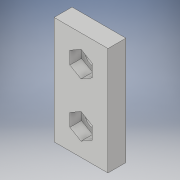
# Autodesk Inventor part: КВ33.044.002 - ограничитель перемещения по оси Z
Saved by Autodesk Inventor 2019 (Build 230136000, 136)
## iProperties
Created: 2019-11-29
Part Number: КВ33.044.002 - ограничитель перемещения по оси Z
Material: Типовые
Document SubType Name: Modeling
Designer: Петров Иван
Density: 1 g/cm^3
Appearance: По умолчанию
Author: Петров Иван
Autodesk Inventor part; units mm, degrees
(part 1 of 2)
ref_plane "YZ Plane" through (0, 0, 0) normal (1, 0, 0) x (0, 1, 0)
ref_plane "XZ Plane" through (0, 0, 0) normal (0, 1, 0) x (-1, 0, 0)
ref_plane "XY Plane" through (0, 0, 0) normal (0, 0, 1) x (1, 0, 0)
sketch "Эскиз1" plane through (0, 0, 0) normal (0, 0, 1) x (1, 0, 0)
  line L0 (-15, -30) -> (15, -30)
  line L1 (15, -30) -> (15, 30)
  line L2 (15, 30) -> (-15, 30)
  line L3 (-15, 30) -> (-15, -30)
  line L4 (-15, -30) -> (15, 30) construction
  line L5 (15, -30) -> (-15, 30) construction
  line L6 (0, 0) -> (0, 15)
  circle A0 centre (0, 15) radius 4.1
  line L7 (0, 0) -> (0, -15)
  circle A1 centre (0, -15) radius 4.1
  dimension "d0" = 30
  dimension "d1" = 60
  dimension "d2" = 15
  dimension "d3" = 8.2
  dimension "d4" = 15
  dimension "d5" = 8.2
  constraints: 16 end point, 2 centre point, 2 coincident, 2 midpoint, 2 parallel, 2 vertical, 1 horizontal, 1 perpendicular
  measures "d0" distance of L2.end L1.end
  measures "d1" distance of L1.end L0.end
  measures "d2" distance of L6.start L6.end
  measures "d3" diameter of A0
  measures "d4" distance of L6.start L7.end
  measures "d5" diameter of A1
extrude "Выдавливание1" add sketch "Эскиз1" along normal blind 10
sketch "Эскиз2" plane through (0, 0, 10) normal (0, 0, 1) x (1, 0, 0)
  circle A0 centre (0, 15) radius 4.1 projected
  line L0 (0, 22.15) -> (6.1921, 18.575)
  line L1 (6.1921, 18.575) -> (6.1921, 11.425)
  line L2 (6.1921, 11.425) -> (0, 7.85)
  line L3 (0, 7.85) -> (-6.1921, 11.425)
  line L4 (-6.1921, 11.425) -> (-6.1921, 18.575)
  line L5 (-6.1921, 18.575) -> (0, 22.15)
  point P0 (0, 0)
  dimension "d8" = 14.3
  constraints: 12 end point, 1 coincident, 13 other
  measures "d8" distance of L2.end L0.start
extrude "Выдавливание2" cut sketch "Эскиз2" against normal blind 6.5
mirror "Зеркальное отражение1" about plane through (0, 0, 0) normal (0, 1, 0) of "Выдавливание2"
sketch "Эскиз3" plane through (15, -30, 0) normal (1, 0, 0) x (0, 0, -1)
  arc A0 (-20.0782, 47.7916) -> (-19.9782, 47.8916) centre (-20.0782, 47.8916) ccw
  line L0 (-19.9782, 47.8916) -> (-19.9782, 57.5416)
  arc A1 (-19.9782, 57.5416) -> (-20.0782, 57.6416) centre (-20.0782, 57.5416) ccw
  line L1 (-19.8782, 57.6416) -> (-19.3657, 57.6416)
  line L2 (-19.3657, 57.6416) -> (-19.274, 56.2076)
  arc A2 (-19.274, 56.2076) -> (-15.0825, 56.2076) centre (-17.1782, 56.3416) ccw
  line L3 (-15.0825, 56.2076) -> (-14.9908, 57.6416)
  line L4 (-14.9908, 57.6416) -> (-10.7025, 57.6416)
  arc A3 (-10.6318, 57.6123) -> (-10.7025, 57.6416) centre (-10.7025, 57.5416) ccw
  line L5 (-10.6318, 57.6123) -> (-10.3075, 57.288)
  arc A4 (-10.3075, 57.288) -> (-9.954, 57.1416) centre (-9.954, 57.6416) ccw
  line L6 (-9.954, 57.1416) -> (-0.2782, 57.1416)
  arc A5 (-0.1782, 57.0416) -> (-0.2782, 57.1416) centre (-0.2782, 57.0416) ccw
  line L7 (-0.1782, 57.0416) -> (-0.1782, 47.8916)
  arc A6 (-0.2782, 47.7916) -> (-0.1782, 47.8916) centre (-0.2782, 47.8916) ccw
  line L8 (-0.2782, 47.7916) -> (-3.204, 47.7916)
  arc A7 (-3.204, 47.7916) -> (-3.5575, 47.6451) centre (-3.204, 47.2916) ccw
  line L9 (-3.5575, 47.6451) -> (-3.8818, 47.3209)
  arc A8 (-3.9525, 47.2916) -> (-3.8818, 47.3209) centre (-3.9525, 47.3916) ccw
  line L10 (-3.9525, 47.2916) -> (-6.704, 47.2916)
  arc A9 (-6.7747, 47.3209) -> (-6.704, 47.2916) centre (-6.704, 47.3916) ccw
  line L11 (-6.7747, 47.3209) -> (-7.099, 47.6451)
  arc A10 (-7.099, 47.6451) -> (-7.4525, 47.7916) centre (-7.4525, 47.2916) ccw
  line L12 (-7.4525, 47.7916) -> (-12.704, 47.7916)
  arc A11 (-12.704, 47.7916) -> (-13.0575, 47.6451) centre (-12.704, 47.2916) ccw
  line L13 (-13.0575, 47.6451) -> (-13.3818, 47.3209)
  arc A12 (-13.4525, 47.2916) -> (-13.3818, 47.3209) centre (-13.4525, 47.3916) ccw
  line L14 (-13.4525, 47.2916) -> (-16.204, 47.2916)
  arc A13 (-16.2747, 47.3209) -> (-16.204, 47.2916) centre (-16.204, 47.3916) ccw
  line L15 (-16.2747, 47.3209) -> (-16.599, 47.6451)
  arc A14 (-16.599, 47.6451) -> (-16.9525, 47.7916) centre (-16.9525, 47.2916) ccw
  line L16 (-16.9525, 47.7916) -> (-19.8782, 47.7916)
  arc A15 (-19.9782, 47.8916) -> (-19.8782, 47.7916) centre (-19.8782, 47.8916) ccw
  arc A16 (-19.8782, 57.6416) -> (-19.9782, 57.5416) centre (-19.8782, 57.5416) ccw
  circle A17 centre (-14.8282, 49.8416) radius 1.25
  circle A18 centre (-5.3282, 49.8416) radius 1.25
  line L17 (-4.1549, 52.0916) -> (-4.7716, 53.3916)
  line L18 (-4.7716, 53.3916) -> (-4.7882, 53.3916)
  line L19 (-4.7882, 53.3916) -> (-5.3882, 52.0916)
  line L20 (-5.3882, 52.0916) -> (-5.2614, 52.0916)
  line L21 (-5.2614, 52.0916) -> (-5.0692, 52.5083)
  line L22 (-5.0692, 52.5083) -> (-4.4799, 52.5083)
  line L23 (-4.4799, 52.5083) -> (-4.2823, 52.0916)
  line L24 (-4.2823, 52.0916) -> (-4.1549, 52.0916)
  spline S0 degree 3 poles (-6.9749, 53.028) (-6.9747, 53.0369) (-6.9742, 53.0544) (-6.9701, 53.08) (-6.9639, 53.1048) (-6.955, 53.1286) (-6.9433, 53.1515) (-6.929, 53.1732) (-6.9125, 53.1943) (-6.8934, 53.214) (-6.8725, 53.2321) (-6.8503, 53.2481) (-6.8269, 53.2615) (-6.8023, 53.2725) (-6.7766, 53.2811) (-6.7497, 53.2871) (-6.7217, 53.2908) (-6.7026, 53.2913) (-6.6929, 53.2916) knots 0 0 0 0 0.061965 0.122122 0.180988 0.239933 0.299906 0.359989 0.421776 0.486576 0.551535 0.615018 0.677259 0.73973 0.80305 0.866495 0.931973 1 1 1 1
  spline S1 degree 3 poles (-6.6929, 53.2916) (-6.6827, 53.2913) (-6.6627, 53.2908) (-6.6334, 53.2872) (-6.6055, 53.2809) (-6.5788, 53.2722) (-6.5533, 53.2613) (-6.5292, 53.2477) (-6.5066, 53.2314) (-6.4852, 53.213) (-6.4656, 53.1924) (-6.4484, 53.1696) (-6.4333, 53.1447) (-6.4201, 53.1181) (-6.4095, 53.0892) (-6.4013, 53.0584) (-6.3948, 53.0257) (-6.3927, 53.0032) (-6.3916, 52.9916) knots 0 0 0 0 0.064439 0.126547 0.186887 0.245878 0.304041 0.362191 0.420976 0.48066 0.5406 0.600689 0.661936 0.724443 0.789038 0.856314 0.926352 1 1 1 1
  line L25 (-6.3916, 52.9916) -> (-6.2749, 52.9916)
  spline S2 degree 3 poles (-6.2749, 52.9916) (-6.2757, 53.0071) (-6.2772, 53.0375) (-6.2842, 53.0818) (-6.2942, 53.1241) (-6.3083, 53.1642) (-6.3259, 53.2023) (-6.347, 53.2384) (-6.3719, 53.2722) (-6.4002, 53.3034) (-6.431, 53.3321) (-6.4641, 53.3568) (-6.499, 53.3778) (-6.5354, 53.3952) (-6.5738, 53.4084) (-6.6139, 53.4181) (-6.6558, 53.424) (-6.6843, 53.4246) (-6.6989, 53.4249) knots 0 0 0 0 0.068791 0.135103 0.198979 0.261904 0.323495 0.385195 0.446969 0.509765 0.572251 0.633405 0.693251 0.752583 0.812579 0.873275 0.93555 1 1 1 1
  spline S3 degree 3 poles (-6.6989, 53.4249) (-6.7131, 53.4246) (-6.7411, 53.4239) (-6.782, 53.4183) (-6.8209, 53.4095) (-6.8578, 53.3971) (-6.8924, 53.3805) (-6.9248, 53.3605) (-6.9556, 53.3374) (-6.9833, 53.3102) (-7.0088, 53.2811) (-7.0307, 53.2501) (-7.0495, 53.2181) (-7.0652, 53.1848) (-7.0767, 53.1499) (-7.0855, 53.114) (-7.0904, 53.0766) (-7.0912, 53.0513) (-7.0916, 53.0385) knots 0 0 0 0 0.069475 0.136517 0.200789 0.26383 0.325735 0.387291 0.449509 0.512968 0.576275 0.63758 0.697903 0.757172 0.816599 0.876653 0.93729 1 1 1 1
  spline S4 degree 3 poles (-7.0916, 53.0385) (-7.0909, 53.0204) (-7.0897, 52.9845) (-7.079, 52.9317) (-7.0624, 52.8806) (-7.0423, 52.8395) (-7.0221, 52.8063) (-7.0039, 52.779) (-6.9825, 52.7497) (-6.9577, 52.7183) (-6.9301, 52.6847) (-6.8992, 52.6488) (-6.865, 52.6111) (-6.841, 52.5854) (-6.8286, 52.5721) knots 0 0 0 0 0.098702 0.195672 0.292422 0.391343 0.444462 0.504229 0.570352 0.642546 0.722288 0.807921 0.90047 1 1 1 1
  line L26 (-6.8286, 52.5721) -> (-6.5033, 52.2249)
  line L27 (-6.5033, 52.2249) -> (-7.1082, 52.2249)
  line L28 (-7.1082, 52.2249) -> (-7.1082, 52.0916)
  line L29 (-7.1082, 52.0916) -> (-6.2249, 52.0916)
  line L30 (-6.2249, 52.0916) -> (-6.7291, 52.6296)
  spline S5 degree 3 poles (-6.7291, 52.6296) (-6.7413, 52.6424) (-6.7649, 52.667) (-6.7983, 52.703) (-6.8282, 52.7363) (-6.855, 52.767) (-6.8779, 52.7954) (-6.8983, 52.8208) (-6.9147, 52.8441) (-6.9324, 52.8711) (-6.9495, 52.9041) (-6.9643, 52.9444) (-6.9733, 52.9859) (-6.9744, 53.0139) (-6.9749, 53.028) knots 0 0 0 0 0.110803 0.212829 0.306101 0.390647 0.466924 0.534481 0.593587 0.644557 0.7362 0.825024 0.911986 1 1 1 1
  line L31 (-7.4849, 52.7416) -> (-7.6182, 53.3916)
  line L32 (-7.6182, 53.3916) -> (-8.1516, 53.3916)
  line L33 (-8.1516, 53.3916) -> (-8.1516, 53.2583)
  line L34 (-8.1516, 53.2583) -> (-7.7094, 53.2583)
  line L35 (-7.7094, 53.2583) -> (-7.6393, 52.9163)
  spline S6 degree 3 poles (-7.6393, 52.9163) (-7.6531, 52.9201) (-7.6798, 52.9275) (-7.7191, 52.9357) (-7.7565, 52.9406) (-7.7807, 52.9413) (-7.7925, 52.9416) knots 0 0 0 0 0.275068 0.532901 0.773973 1 1 1 1
  spline S7 degree 3 poles (-7.7925, 52.9416) (-7.807, 52.9413) (-7.8355, 52.9407) (-7.8773, 52.9347) (-7.9171, 52.9254) (-7.955, 52.9123) (-7.991, 52.8957) (-8.0247, 52.8748) (-8.0567, 52.8505) (-8.0864, 52.8225) (-8.1134, 52.7917) (-8.1371, 52.7586) (-8.1572, 52.7235) (-8.1734, 52.686) (-8.1863, 52.6467) (-8.1949, 52.605) (-8.2006, 52.5614) (-8.2012, 52.5315) (-8.2016, 52.5163) knots 0 0 0 0 0.065808 0.129394 0.190894 0.251281 0.310815 0.370371 0.430768 0.492881 0.555104 0.616067 0.677256 0.73826 0.800762 0.864778 0.931045 1 1 1 1
  spline S8 degree 3 poles (-8.2016, 52.5163) (-8.2013, 52.5057) (-8.2008, 52.4847) (-8.1983, 52.4534) (-8.1935, 52.4228) (-8.1871, 52.3929) (-8.1787, 52.3637) (-8.1686, 52.3351) (-8.1562, 52.3073) (-8.1426, 52.2801) (-8.1272, 52.254) (-8.1102, 52.2296) (-8.0923, 52.2066) (-8.0729, 52.1851) (-8.0521, 52.1653) (-8.0299, 52.1471) (-8.0066, 52.1302) (-7.9819, 52.1153) (-7.9562, 52.1016) (-7.9292, 52.0903) (-7.9016, 52.0802) (-7.8728, 52.0722) (-7.8431, 52.0659) (-7.8123, 52.0617) (-7.7805, 52.0585) (-7.759, 52.0584) (-7.7482, 52.0583) knots 0 0 0 0 0.044014 0.087434 0.130118 0.172554 0.214555 0.256298 0.298438 0.340849 0.382715 0.423924 0.464246 0.504074 0.543862 0.583567 0.623094 0.663229 0.703551 0.743938 0.784541 0.82575 0.867757 0.910745 0.954914 1 1 1 1
  spline S9 degree 3 poles (-7.7482, 52.0583) (-7.7352, 52.0585) (-7.7098, 52.059) (-7.6724, 52.0643) (-7.6365, 52.0719) (-7.6023, 52.0832) (-7.5694, 52.0975) (-7.5385, 52.1155) (-7.5085, 52.1359) (-7.4808, 52.16) (-7.4552, 52.1864) (-7.4322, 52.215) (-7.4117, 52.2453) (-7.3941, 52.2776) (-7.379, 52.3117) (-7.3672, 52.3478) (-7.3577, 52.3856) (-7.3536, 52.4117) (-7.3516, 52.4249) knots 0 0 0 0 0.065421 0.128708 0.190236 0.250724 0.310637 0.370766 0.431615 0.493523 0.555883 0.617342 0.678668 0.740711 0.802985 0.866803 0.932347 1 1 1 1
  line L36 (-7.3516, 52.4249) -> (-7.4682, 52.4249)
  spline S10 degree 3 poles (-7.4682, 52.4249) (-7.4711, 52.4125) (-7.4766, 52.3887) (-7.4887, 52.3552) (-7.5035, 52.3254) (-7.5212, 52.2988) (-7.5422, 52.2756) (-7.5661, 52.255) (-7.593, 52.2363) (-7.6229, 52.2208) (-7.6544, 52.2075) (-7.6873, 52.1987) (-7.7209, 52.1925) (-7.7436, 52.1919) (-7.755, 52.1916) knots 0 0 0 0 0.094687 0.181994 0.264377 0.34218 0.418618 0.496509 0.577369 0.661511 0.746733 0.831258 0.915206 1 1 1 1
  spline S11 degree 3 poles (-7.755, 52.1916) (-7.7661, 52.1919) (-7.788, 52.1925) (-7.8202, 52.1971) (-7.8514, 52.2042) (-7.8811, 52.2149) (-7.9099, 52.2278) (-7.9371, 52.2444) (-7.9634, 52.2635) (-7.9881, 52.2854) (-8.0107, 52.3096) (-8.0306, 52.3354) (-8.0473, 52.3629) (-8.0613, 52.3917) (-8.0719, 52.422) (-8.0795, 52.4538) (-8.084, 52.487) (-8.0846, 52.5097) (-8.0849, 52.5213) knots 0 0 0 0 0.064207 0.126425 0.18768 0.248216 0.308305 0.369661 0.431699 0.495947 0.559758 0.622295 0.683911 0.745092 0.80674 0.869087 0.93329 1 1 1 1
  spline S12 degree 3 poles (-8.0849, 52.5213) (-8.0847, 52.5317) (-8.0842, 52.5521) (-8.0803, 52.582) (-8.0735, 52.6102) (-8.064, 52.637) (-8.052, 52.6624) (-8.0374, 52.6863) (-8.0198, 52.7085) (-7.9997, 52.7289) (-7.9777, 52.7478) (-7.9534, 52.7639) (-7.9273, 52.7775) (-7.8997, 52.7891) (-7.87, 52.7975) (-7.8388, 52.8038) (-7.8057, 52.8075) (-7.783, 52.808) (-7.7714, 52.8083) knots 0 0 0 0 0.065351 0.127916 0.18836 0.247216 0.30563 0.36377 0.422661 0.482687 0.5433 0.604118 0.664965 0.727413 0.791468 0.858055 0.927037 1 1 1 1
  spline S13 degree 3 poles (-7.7714, 52.8083) (-7.7613, 52.808) (-7.7405, 52.8076) (-7.7086, 52.8043) (-7.675, 52.799) (-7.64, 52.7917) (-7.6034, 52.7822) (-7.5652, 52.7708) (-7.5255, 52.7572) (-7.4987, 52.7469) (-7.4849, 52.7416) knots 0 0 0 0 0.102203 0.211023 0.3251 0.446502 0.573788 0.708901 0.850358 1 1 1 1
  line L37 (-10.9316, 52.0916) -> (-11.5482, 53.3916)
  line L38 (-11.5482, 53.3916) -> (-11.5649, 53.3916)
  line L39 (-11.5649, 53.3916) -> (-12.1649, 52.0916)
  line L40 (-12.1649, 52.0916) -> (-12.0381, 52.0916)
  line L41 (-12.0381, 52.0916) -> (-11.8459, 52.5083)
  line L42 (-11.8459, 52.5083) -> (-11.2566, 52.5083)
  line L43 (-11.2566, 52.5083) -> (-11.0589, 52.0916)
  line L44 (-11.0589, 52.0916) -> (-10.9316, 52.0916)
  spline S14 degree 3 poles (-12.4416, 52.7491) (-12.4422, 52.7725) (-12.4433, 52.8185) (-12.4529, 52.886) (-12.4685, 52.9507) (-12.4905, 53.0125) (-12.5185, 53.0716) (-12.5531, 53.1276) (-12.5938, 53.1809) (-12.6404, 53.2307) (-12.6915, 53.2762) (-12.7462, 53.3162) (-12.8044, 53.3496) (-12.8655, 53.3774) (-12.93, 53.3988) (-12.9976, 53.4138) (-13.0683, 53.4231) (-13.1165, 53.4243) (-13.1411, 53.4249) knots 0 0 0 0 0.064558 0.127014 0.187955 0.248014 0.307748 0.368235 0.42947 0.492743 0.556258 0.618217 0.679655 0.741246 0.803415 0.866815 0.932328 1 1 1 1
  spline S15 degree 3 poles (-13.1411, 53.4249) (-13.156, 53.4247) (-13.1856, 53.4244) (-13.2293, 53.4209) (-13.2719, 53.4152) (-13.3133, 53.4073) (-13.3539, 53.3976) (-13.3932, 53.3849) (-13.4315, 53.3704) (-13.4685, 53.3537) (-13.5041, 53.335) (-13.5383, 53.3144) (-13.5708, 53.292) (-13.6018, 53.268) (-13.6308, 53.2418) (-13.6587, 53.2143) (-13.6844, 53.1845) (-13.7003, 53.1635) (-13.7082, 53.153) knots 0 0 0 0 0.068548 0.135683 0.201215 0.265682 0.329267 0.392395 0.45507 0.517127 0.57879 0.63974 0.700192 0.759806 0.819628 0.879355 0.939512 1 1 1 1
  line L45 (-13.7082, 53.153) -> (-13.6062, 53.0749)
  spline S16 degree 3 poles (-13.6062, 53.0749) (-13.5989, 53.0836) (-13.5844, 53.1008) (-13.5611, 53.125) (-13.5369, 53.1477) (-13.5117, 53.169) (-13.485, 53.1881) (-13.4576, 53.206) (-13.4289, 53.2221) (-13.3892, 53.2416) (-13.3374, 53.2619) (-13.2721, 53.279) (-13.2039, 53.2898) (-13.1574, 53.291) (-13.1338, 53.2916) knots 0 0 0 0 0.063163 0.125475 0.187121 0.248294 0.309295 0.36985 0.430973 0.492456 0.616148 0.740844 0.868183 1 1 1 1
  spline S17 degree 3 poles (-13.1338, 53.2916) (-13.1207, 53.2914) (-13.0948, 53.2911) (-13.0563, 53.2872) (-13.0185, 53.2817) (-12.9815, 53.2734) (-12.9452, 53.2631) (-12.9095, 53.2506) (-12.8749, 53.2353) (-12.8409, 53.2183) (-12.8083, 53.1991) (-12.7774, 53.1782) (-12.7485, 53.1558) (-12.7213, 53.1318) (-12.696, 53.1063) (-12.6727, 53.079) (-12.6514, 53.0501) (-12.6319, 53.0199) (-12.6143, 52.9885) (-12.5996, 52.9558) (-12.5866, 52.9223) (-12.5763, 52.8877) (-12.5682, 52.8522) (-12.5626, 52.8158) (-12.5587, 52.7784) (-12.5584, 52.7531) (-12.5582, 52.7403) knots 0 0 0 0 0.043955 0.087502 0.130463 0.172752 0.215403 0.25765 0.300153 0.343121 0.385925 0.427686 0.468818 0.509492 0.549883 0.58998 0.630405 0.670869 0.711384 0.751627 0.791776 0.832459 0.873319 0.914543 0.956924 1 1 1 1
  spline S18 degree 3 poles (-12.5582, 52.7403) (-12.5587, 52.7211) (-12.5596, 52.6833) (-12.5678, 52.6281) (-12.5803, 52.5752) (-12.5989, 52.5249) (-12.6219, 52.4766) (-12.651, 52.4312) (-12.6846, 52.388) (-12.7234, 52.3479) (-12.7659, 52.3113) (-12.8114, 52.2791) (-12.86, 52.2522) (-12.9111, 52.2299) (-12.9649, 52.2127) (-13.0215, 52.2006) (-13.0808, 52.1927) (-13.1212, 52.192) (-13.1418, 52.1916) knots 0 0 0 0 0.064323 0.12629 0.186726 0.246146 0.305576 0.365429 0.426326 0.48884 0.551725 0.613919 0.675484 0.737334 0.800229 0.864502 0.931041 1 1 1 1
  spline S19 degree 3 poles (-13.1418, 52.1916) (-13.1645, 52.1922) (-13.2092, 52.1934) (-13.2747, 52.2039) (-13.3374, 52.2209) (-13.3973, 52.2446) (-13.4543, 52.2755) (-13.5084, 52.3129) (-13.5596, 52.3572) (-13.5904, 52.391) (-13.6062, 52.4083) knots 0 0 0 0 0.128515 0.252949 0.374755 0.49594 0.617181 0.740909 0.867811 1 1 1 1
  line L46 (-13.6062, 52.4083) -> (-13.7082, 52.3309)
  spline S20 degree 3 poles (-13.7082, 52.3309) (-13.7, 52.3203) (-13.6836, 52.2992) (-13.6571, 52.2693) (-13.6291, 52.2413) (-13.5995, 52.2153) (-13.5687, 52.1907) (-13.536, 52.1683) (-13.5018, 52.1477) (-13.4664, 52.1289) (-13.4297, 52.1123) (-13.3919, 52.098) (-13.3529, 52.0857) (-13.3129, 52.0756) (-13.2718, 52.0676) (-13.2297, 52.0624) (-13.1865, 52.0587) (-13.1574, 52.0584) (-13.1426, 52.0583) knots 0 0 0 0 0.061674 0.123053 0.183475 0.243727 0.304279 0.364863 0.425946 0.487391 0.54922 0.611144 0.673529 0.736961 0.800785 0.866013 0.932101 1 1 1 1
  spline S21 degree 3 poles (-13.1426, 52.0583) (-13.1286, 52.0584) (-13.101, 52.0585) (-13.0602, 52.0617) (-13.0204, 52.0659) (-12.9819, 52.0723) (-12.9443, 52.0799) (-12.9081, 52.09) (-12.8728, 52.1013) (-12.8387, 52.1147) (-12.8056, 52.1297) (-12.7737, 52.1467) (-12.743, 52.1656) (-12.7132, 52.1858) (-12.6848, 52.2081) (-12.6574, 52.2321) (-12.631, 52.2578) (-12.6146, 52.2763) (-12.6064, 52.2856) knots 0 0 0 0 0.069663 0.13775 0.203917 0.26878 0.332414 0.394754 0.45618 0.516996 0.577396 0.637198 0.696999 0.756756 0.816554 0.876948 0.938132 1 1 1 1
  spline S22 degree 3 poles (-12.6064, 52.2856) (-12.5933, 52.3018) (-12.5671, 52.3339) (-12.5336, 52.386) (-12.505, 52.4404) (-12.4818, 52.4974) (-12.4637, 52.5569) (-12.4511, 52.6188) (-12.443, 52.6831) (-12.442, 52.7269) (-12.4416, 52.7491) knots 0 0 0 0 0.124329 0.247156 0.36878 0.490734 0.613614 0.738958 0.867311 1 1 1 1
  line L47 (-15.5142, 53.3416) -> (-15.3014, 53.3416)
  line L48 (-15.1139, 52.2416) -> (-15.5142, 53.3416)
  line L49 (-15.6139, 52.2416) -> (-15.1139, 52.2416)
  line L50 (-16.0142, 53.3416) -> (-15.6139, 52.2416)
  line L51 (-16.2271, 53.3416) -> (-16.0142, 53.3416)
  line L52 (-15.8267, 52.2416) -> (-16.2271, 53.3416)
  line L53 (-16.0267, 52.2416) -> (-15.8267, 52.2416)
  line L54 (-15.9539, 52.0416) -> (-16.0267, 52.2416)
  line L55 (-14.8282, 52.0416) -> (-15.9539, 52.0416)
  line L56 (-15.3014, 53.3416) -> (-14.8282, 52.0416)
  line L57 (-10.1382, 52.0916) -> (-10.1216, 52.0916)
  line L58 (-10.1216, 52.0916) -> (-9.5716, 53.3916)
  line L59 (-9.5716, 53.3916) -> (-9.6966, 53.3916)
  line L60 (-9.6966, 53.3916) -> (-10.1299, 52.3671)
  line L61 (-10.1299, 52.3671) -> (-10.5632, 53.3916)
  line L62 (-10.5632, 53.3916) -> (-10.6882, 53.3916)
  line L63 (-10.6882, 53.3916) -> (-10.1382, 52.0916)
  spline S23 degree 3 poles (-9.3282, 52.7411) (-9.328, 52.7212) (-9.3275, 52.6824) (-9.3251, 52.6258) (-9.3203, 52.5723) (-9.3142, 52.5219) (-9.3059, 52.4747) (-9.2957, 52.4306) (-9.2843, 52.3894) (-9.2702, 52.3514) (-9.2548, 52.3161) (-9.2381, 52.2832) (-9.2202, 52.2523) (-9.2006, 52.2237) (-9.1798, 52.1972) (-9.1573, 52.1732) (-9.1336, 52.1512) (-9.1086, 52.1317) (-9.0824, 52.1146) (-9.0557, 52.0993) (-9.0279, 52.0869) (-8.9997, 52.0763) (-8.9707, 52.0682) (-8.9409, 52.0626) (-8.9105, 52.0587) (-8.8899, 52.0584) (-8.8795, 52.0583) knots 0 0 0 0 0.065063 0.126773 0.185516 0.240765 0.29298 0.34225 0.388919 0.432776 0.474628 0.514775 0.553606 0.591426 0.628028 0.663804 0.698984 0.733591 0.767628 0.801208 0.834264 0.866981 0.89972 0.932702 0.966176 1 1 1 1
  spline S24 degree 3 poles (-8.8795, 52.0583) (-8.8693, 52.0584) (-8.8491, 52.0588) (-8.8191, 52.0623) (-8.79, 52.068) (-8.7617, 52.0759) (-8.734, 52.0857) (-8.7072, 52.0984) (-8.6811, 52.113) (-8.6557, 52.1296) (-8.6316, 52.1487) (-8.6085, 52.1698) (-8.5871, 52.1934) (-8.5672, 52.2192) (-8.5482, 52.2469) (-8.5308, 52.277) (-8.5147, 52.3092) (-8.5, 52.3439) (-8.4869, 52.3815) (-8.4754, 52.4224) (-8.4663, 52.467) (-8.4585, 52.515) (-8.4522, 52.5665) (-8.4479, 52.6216) (-8.4453, 52.6802) (-8.445, 52.7204) (-8.4449, 52.7411) knots 0 0 0 0 0.033787 0.066622 0.099285 0.131361 0.163585 0.196104 0.228902 0.262158 0.295991 0.330218 0.36506 0.400951 0.43762 0.475708 0.515381 0.556414 0.599765 0.646424 0.696431 0.749782 0.806573 0.867436 0.931887 1 1 1 1
  spline S25 degree 3 poles (-8.4449, 52.7411) (-8.445, 52.7619) (-8.4453, 52.8024) (-8.4479, 52.8614) (-8.4523, 52.9167) (-8.4583, 52.9684) (-8.4656, 53.0164) (-8.4753, 53.0607) (-8.4864, 53.1014) (-8.4992, 53.1387) (-8.5137, 53.1731) (-8.5294, 53.2052) (-8.5471, 53.235) (-8.5657, 53.2629) (-8.5859, 53.2885) (-8.6072, 53.3121) (-8.6304, 53.3333) (-8.6547, 53.3525) (-8.6803, 53.3694) (-8.7065, 53.3843) (-8.7336, 53.397) (-8.7614, 53.407) (-8.7899, 53.4152) (-8.8191, 53.4209) (-8.8491, 53.4244) (-8.8693, 53.4247) (-8.8795, 53.4249) knots 0 0 0 0 0.068595 0.133246 0.194313 0.251279 0.304513 0.354235 0.400481 0.443411 0.484015 0.523252 0.561042 0.5979 0.633518 0.668314 0.702496 0.736685 0.770293 0.803437 0.835913 0.86846 0.900847 0.933467 0.966258 1 1 1 1
  spline S26 degree 3 poles (-8.8795, 53.4249) (-8.8899, 53.4247) (-8.9104, 53.4244) (-8.9408, 53.4209) (-8.9705, 53.4152) (-8.9994, 53.407) (-9.0277, 53.3969) (-9.0551, 53.3843) (-9.082, 53.3695) (-9.1077, 53.3522) (-9.1327, 53.3329) (-9.1562, 53.3111) (-9.1784, 53.287) (-9.1995, 53.2608) (-9.2188, 53.2321) (-9.2372, 53.2013) (-9.2537, 53.168) (-9.2696, 53.1327) (-9.2833, 53.0943) (-9.2956, 53.0532) (-9.3056, 53.0087) (-9.3139, 52.9613) (-9.3204, 52.9106) (-9.3251, 52.8569) (-9.3275, 52.7999) (-9.328, 52.761) (-9.3282, 52.7411) knots 0 0 0 0 0.033788 0.067194 0.099862 0.132567 0.165151 0.197913 0.231319 0.265083 0.299255 0.334399 0.369943 0.406284 0.444064 0.482998 0.523354 0.565537 0.609613 0.656391 0.705885 0.758325 0.813832 0.872795 0.934722 1 1 1 1
  line L64 (-3.1782, 52.7416) -> (-3.3116, 53.3916)
  line L65 (-3.3116, 53.3916) -> (-3.8449, 53.3916)
  line L66 (-3.8449, 53.3916) -> (-3.8449, 53.2583)
  line L67 (-3.8449, 53.2583) -> (-3.4027, 53.2583)
  line L68 (-3.4027, 53.2583) -> (-3.3327, 52.9163)
  spline S27 degree 3 poles (-3.3327, 52.9163) (-3.3464, 52.9201) (-3.3731, 52.9275) (-3.4125, 52.9357) (-3.4498, 52.9406) (-3.4741, 52.9413) (-3.4858, 52.9416) knots 0 0 0 0 0.275068 0.532901 0.773973 1 1 1 1
  spline S28 degree 3 poles (-3.4858, 52.9416) (-3.5003, 52.9413) (-3.5289, 52.9407) (-3.5706, 52.9347) (-3.6105, 52.9254) (-3.6484, 52.9123) (-3.6843, 52.8957) (-3.7181, 52.8748) (-3.7501, 52.8505) (-3.7798, 52.8225) (-3.8067, 52.7917) (-3.8304, 52.7586) (-3.8505, 52.7235) (-3.8667, 52.686) (-3.8796, 52.6467) (-3.8882, 52.605) (-3.8939, 52.5614) (-3.8946, 52.5315) (-3.8949, 52.5163) knots 0 0 0 0 0.065808 0.129394 0.190894 0.251281 0.310815 0.370371 0.430768 0.492881 0.555104 0.616067 0.677256 0.73826 0.800762 0.864778 0.931045 1 1 1 1
  spline S29 degree 3 poles (-3.8949, 52.5163) (-3.8947, 52.5057) (-3.8942, 52.4847) (-3.8917, 52.4534) (-3.8869, 52.4228) (-3.8804, 52.3929) (-3.872, 52.3637) (-3.8619, 52.3351) (-3.8495, 52.3073) (-3.8359, 52.2801) (-3.8206, 52.254) (-3.8036, 52.2296) (-3.7856, 52.2066) (-3.7663, 52.1851) (-3.7454, 52.1653) (-3.7232, 52.1471) (-3.7, 52.1302) (-3.6752, 52.1153) (-3.6495, 52.1016) (-3.6225, 52.0903) (-3.5949, 52.0802) (-3.5662, 52.0722) (-3.5364, 52.0659) (-3.5056, 52.0617) (-3.4739, 52.0585) (-3.4524, 52.0584) (-3.4415, 52.0583) knots 0 0 0 0 0.044014 0.087434 0.130118 0.172554 0.214555 0.256298 0.298438 0.340849 0.382715 0.423924 0.464246 0.504074 0.543862 0.583567 0.623094 0.663229 0.703551 0.743938 0.784541 0.82575 0.867757 0.910745 0.954914 1 1 1 1
  spline S30 degree 3 poles (-3.4415, 52.0583) (-3.4286, 52.0585) (-3.4031, 52.059) (-3.3657, 52.0643) (-3.3298, 52.0719) (-3.2956, 52.0832) (-3.2628, 52.0975) (-3.2318, 52.1155) (-3.2019, 52.1359) (-3.1742, 52.16) (-3.1485, 52.1864) (-3.1255, 52.215) (-3.105, 52.2453) (-3.0874, 52.2776) (-3.0723, 52.3117) (-3.0605, 52.3478) (-3.051, 52.3856) (-3.047, 52.4117) (-3.0449, 52.4249) knots 0 0 0 0 0.065421 0.128708 0.190236 0.250724 0.310637 0.370766 0.431615 0.493523 0.555883 0.617342 0.678668 0.740711 0.802985 0.866803 0.932347 1 1 1 1
  line L69 (-3.0449, 52.4249) -> (-3.1616, 52.4249)
  spline S31 degree 3 poles (-3.1616, 52.4249) (-3.1644, 52.4125) (-3.17, 52.3887) (-3.1821, 52.3552) (-3.1969, 52.3254) (-3.2145, 52.2988) (-3.2355, 52.2756) (-3.2595, 52.255) (-3.2863, 52.2363) (-3.3162, 52.2208) (-3.3477, 52.2075) (-3.3807, 52.1987) (-3.4142, 52.1925) (-3.4369, 52.1919) (-3.4483, 52.1916) knots 0 0 0 0 0.094687 0.181994 0.264377 0.34218 0.418618 0.496509 0.577369 0.661511 0.746733 0.831258 0.915206 1 1 1 1
  spline S32 degree 3 poles (-3.4483, 52.1916) (-3.4594, 52.1919) (-3.4813, 52.1925) (-3.5136, 52.1971) (-3.5447, 52.2042) (-3.5744, 52.2149) (-3.6032, 52.2278) (-3.6304, 52.2444) (-3.6567, 52.2635) (-3.6814, 52.2854) (-3.704, 52.3096) (-3.724, 52.3354) (-3.7406, 52.3629) (-3.7546, 52.3917) (-3.7653, 52.422) (-3.7729, 52.4538) (-3.7773, 52.487) (-3.7779, 52.5097) (-3.7782, 52.5213) knots 0 0 0 0 0.064207 0.126425 0.18768 0.248216 0.308305 0.369661 0.431699 0.495947 0.559758 0.622295 0.683911 0.745092 0.80674 0.869087 0.93329 1 1 1 1
  spline S33 degree 3 poles (-3.7782, 52.5213) (-3.778, 52.5317) (-3.7775, 52.5521) (-3.7736, 52.582) (-3.7668, 52.6102) (-3.7574, 52.637) (-3.7454, 52.6624) (-3.7307, 52.6863) (-3.7131, 52.7085) (-3.693, 52.7289) (-3.671, 52.7478) (-3.6467, 52.7639) (-3.6206, 52.7775) (-3.5931, 52.7891) (-3.5634, 52.7975) (-3.5321, 52.8038) (-3.499, 52.8075) (-3.4763, 52.808) (-3.4647, 52.8083) knots 0 0 0 0 0.065351 0.127916 0.18836 0.247216 0.30563 0.36377 0.422661 0.482687 0.5433 0.604118 0.664965 0.727413 0.791468 0.858055 0.927037 1 1 1 1
  spline S34 degree 3 poles (-3.4647, 52.8083) (-3.4546, 52.808) (-3.4338, 52.8076) (-3.4019, 52.8043) (-3.3684, 52.799) (-3.3333, 52.7917) (-3.2967, 52.7822) (-3.2586, 52.7708) (-3.2188, 52.7572) (-3.192, 52.7469) (-3.1782, 52.7416) knots 0 0 0 0 0.102203 0.211023 0.3251 0.446502 0.573788 0.708901 0.850358 1 1 1 1
  line L70 (0, 60) -> (-10, 60) projected
  line L71 (0, 60) -> (-21.0398, 60)
  line L72 (-21.0398, 60) -> (-21.0398, 45.6746)
  line L73 (-21.0398, 45.6746) -> (0, 45.6746)
  line L74 (0, 45.6746) -> (0, 60)
  point P0 (0, 30)
  constraints: 148 end point, 34 point on circle, 19 centre point, 4 symmetric about line, 2 parallel, 1 horizontal, 1 perpendicular, 74 other
extrude "Выдавливание3" [suppressed]
sketch "Эскиз4" plane through (15, -30, 0) normal (1, 0, 0) x (0, 0, -1)
  arc A0 (-20.0782, 47.7916) -> (-19.9782, 47.8916) centre (-20.0782, 47.8916) ccw
  line L0 (-19.9782, 47.8916) -> (-19.9782, 57.5416)
  arc A1 (-19.9782, 57.5416) -> (-20.0782, 57.6416) centre (-20.0782, 57.5416) ccw
  line L1 (-14.8282, 52.0416) -> (-15.9539, 52.0416)
  line L2 (-16.0267, 52.2416) -> (-15.8267, 52.2416)
  line L3 (-15.9539, 52.0416) -> (-16.0267, 52.2416)
  line L4 (-15.6139, 52.2416) -> (-15.1139, 52.2416)
  line L5 (-15.3014, 53.3416) -> (-14.8282, 52.0416)
  line L6 (-15.1139, 52.2416) -> (-15.5142, 53.3416)
  line L7 (-15.8267, 52.2416) -> (-16.2271, 53.3416)
  line L8 (-16.0142, 53.3416) -> (-15.6139, 52.2416)
  line L9 (-15.5142, 53.3416) -> (-15.3014, 53.3416)
  line L10 (-16.2271, 53.3416) -> (-16.0142, 53.3416)
  arc A2 (-19.274, 56.2076) -> (-15.0825, 56.2076) centre (-17.1782, 56.3416) ccw
  line L11 (-19.3657, 57.6416) -> (-19.274, 56.2076)
  line L12 (-19.8782, 57.6416) -> (-19.3657, 57.6416)
  line L13 (-4.2823, 52.0916) -> (-4.1549, 52.0916)
  line L14 (-4.4799, 52.5083) -> (-4.2823, 52.0916)
  line L15 (-4.7716, 53.3916) -> (-4.7882, 53.3916)
  line L16 (-5.0692, 52.5083) -> (-4.4799, 52.5083)
  line L17 (-5.2614, 52.0916) -> (-5.0692, 52.5083)
  line L18 (-5.3882, 52.0916) -> (-5.2614, 52.0916)
  line L19 (-4.7882, 53.3916) -> (-5.3882, 52.0916)
  spline S0 degree 3 poles (-6.6929, 53.2916) (-6.6827, 53.2913) (-6.6627, 53.2908) (-6.6334, 53.2872) (-6.6055, 53.2809) (-6.5788, 53.2722) (-6.5533, 53.2613) (-6.5292, 53.2477) (-6.5066, 53.2314) (-6.4852, 53.213) (-6.4656, 53.1924) (-6.4484, 53.1696) (-6.4333, 53.1447) (-6.4201, 53.1181) (-6.4095, 53.0892) (-6.4013, 53.0584) (-6.3948, 53.0257) (-6.3927, 53.0032) (-6.3916, 52.9916) knots 0 0 0 0 0.064439 0.126547 0.186887 0.245878 0.304041 0.362191 0.420976 0.48066 0.5406 0.600689 0.661936 0.724443 0.789038 0.856314 0.926352 1 1 1 1
  line L20 (-4.1549, 52.0916) -> (-4.7716, 53.3916)
  line L21 (-12.0381, 52.0916) -> (-11.8459, 52.5083)
  line L22 (-11.5649, 53.3916) -> (-12.1649, 52.0916)
  line L23 (-11.5482, 53.3916) -> (-11.5649, 53.3916)
  line L24 (-11.8459, 52.5083) -> (-11.2566, 52.5083)
  line L25 (-10.9316, 52.0916) -> (-11.5482, 53.3916)
  line L26 (-12.1649, 52.0916) -> (-12.0381, 52.0916)
  line L27 (-9.5716, 53.3916) -> (-9.6966, 53.3916)
  line L28 (-9.6966, 53.3916) -> (-10.1299, 52.3671)
  line L29 (-10.1382, 52.0916) -> (-10.1216, 52.0916)
  line L30 (-10.1299, 52.3671) -> (-10.5632, 53.3916)
  line L31 (-10.5632, 53.3916) -> (-10.6882, 53.3916)
  line L32 (-10.6882, 53.3916) -> (-10.1382, 52.0916)
  line L33 (-11.0589, 52.0916) -> (-10.9316, 52.0916)
  line L34 (-11.2566, 52.5083) -> (-11.0589, 52.0916)
  line L35 (-10.1216, 52.0916) -> (-9.5716, 53.3916)
  circle A3 centre (-14.8282, 49.8416) radius 1.25
  arc A4 (-16.599, 47.6451) -> (-16.9525, 47.7916) centre (-16.9525, 47.2916) ccw
  line L36 (-16.2747, 47.3209) -> (-16.599, 47.6451)
  arc A5 (-16.2747, 47.3209) -> (-16.204, 47.2916) centre (-16.204, 47.3916) ccw
  line L37 (-13.4525, 47.2916) -> (-16.204, 47.2916)
  arc A6 (-13.4525, 47.2916) -> (-13.3818, 47.3209) centre (-13.4525, 47.3916) ccw
  arc A7 (-12.704, 47.7916) -> (-13.0575, 47.6451) centre (-12.704, 47.2916) ccw
  line L38 (-13.0575, 47.6451) -> (-13.3818, 47.3209)
  spline S1 degree 3 poles (-8.8795, 53.4249) (-8.8899, 53.4247) (-8.9104, 53.4244) (-8.9408, 53.4209) (-8.9705, 53.4152) (-8.9994, 53.407) (-9.0277, 53.3969) (-9.0551, 53.3843) (-9.082, 53.3695) (-9.1077, 53.3522) (-9.1327, 53.3329) (-9.1562, 53.3111) (-9.1784, 53.287) (-9.1995, 53.2608) (-9.2188, 53.2321) (-9.2372, 53.2013) (-9.2537, 53.168) (-9.2696, 53.1327) (-9.2833, 53.0943) (-9.2956, 53.0532) (-9.3056, 53.0087) (-9.3139, 52.9613) (-9.3204, 52.9106) (-9.3251, 52.8569) (-9.3275, 52.7999) (-9.328, 52.761) (-9.3282, 52.7411) knots 0 0 0 0 0.033788 0.067194 0.099862 0.132567 0.165151 0.197913 0.231319 0.265083 0.299255 0.334399 0.369943 0.406284 0.444064 0.482998 0.523354 0.565537 0.609613 0.656391 0.705885 0.758325 0.813832 0.872795 0.934722 1 1 1 1
  spline S2 degree 3 poles (-9.3282, 52.7411) (-9.328, 52.7212) (-9.3275, 52.6824) (-9.3251, 52.6258) (-9.3203, 52.5723) (-9.3142, 52.5219) (-9.3059, 52.4747) (-9.2957, 52.4306) (-9.2843, 52.3894) (-9.2702, 52.3514) (-9.2548, 52.3161) (-9.2381, 52.2832) (-9.2202, 52.2523) (-9.2006, 52.2237) (-9.1798, 52.1972) (-9.1573, 52.1732) (-9.1336, 52.1512) (-9.1086, 52.1317) (-9.0824, 52.1146) (-9.0557, 52.0993) (-9.0279, 52.0869) (-8.9997, 52.0763) (-8.9707, 52.0682) (-8.9409, 52.0626) (-8.9105, 52.0587) (-8.8899, 52.0584) (-8.8795, 52.0583) knots 0 0 0 0 0.065063 0.126773 0.185516 0.240765 0.29298 0.34225 0.388919 0.432776 0.474628 0.514775 0.553606 0.591426 0.628028 0.663804 0.698984 0.733591 0.767628 0.801208 0.834264 0.866981 0.89972 0.932702 0.966176 1 1 1 1
  spline S3 degree 3 poles (-8.4449, 52.7411) (-8.445, 52.7619) (-8.4453, 52.8024) (-8.4479, 52.8614) (-8.4523, 52.9167) (-8.4583, 52.9684) (-8.4656, 53.0164) (-8.4753, 53.0607) (-8.4864, 53.1014) (-8.4992, 53.1387) (-8.5137, 53.1731) (-8.5294, 53.2052) (-8.5471, 53.235) (-8.5657, 53.2629) (-8.5859, 53.2885) (-8.6072, 53.3121) (-8.6304, 53.3333) (-8.6547, 53.3525) (-8.6803, 53.3694) (-8.7065, 53.3843) (-8.7336, 53.397) (-8.7614, 53.407) (-8.7899, 53.4152) (-8.8191, 53.4209) (-8.8491, 53.4244) (-8.8693, 53.4247) (-8.8795, 53.4249) knots 0 0 0 0 0.068595 0.133246 0.194313 0.251279 0.304513 0.354235 0.400481 0.443411 0.484015 0.523252 0.561042 0.5979 0.633518 0.668314 0.702496 0.736685 0.770293 0.803437 0.835913 0.86846 0.900847 0.933467 0.966258 1 1 1 1
  spline S4 degree 3 poles (-8.8795, 52.0583) (-8.8693, 52.0584) (-8.8491, 52.0588) (-8.8191, 52.0623) (-8.79, 52.068) (-8.7617, 52.0759) (-8.734, 52.0857) (-8.7072, 52.0984) (-8.6811, 52.113) (-8.6557, 52.1296) (-8.6316, 52.1487) (-8.6085, 52.1698) (-8.5871, 52.1934) (-8.5672, 52.2192) (-8.5482, 52.2469) (-8.5308, 52.277) (-8.5147, 52.3092) (-8.5, 52.3439) (-8.4869, 52.3815) (-8.4754, 52.4224) (-8.4663, 52.467) (-8.4585, 52.515) (-8.4522, 52.5665) (-8.4479, 52.6216) (-8.4453, 52.6802) (-8.445, 52.7204) (-8.4449, 52.7411) knots 0 0 0 0 0.033787 0.066622 0.099285 0.131361 0.163585 0.196104 0.228902 0.262158 0.295991 0.330218 0.36506 0.400951 0.43762 0.475708 0.515381 0.556414 0.599765 0.646424 0.696431 0.749782 0.806573 0.867436 0.931887 1 1 1 1
  line L39 (-8.1516, 53.3916) -> (-8.1516, 53.2583)
  spline S5 degree 3 poles (-8.2016, 52.5163) (-8.2013, 52.5057) (-8.2008, 52.4847) (-8.1983, 52.4534) (-8.1935, 52.4228) (-8.1871, 52.3929) (-8.1787, 52.3637) (-8.1686, 52.3351) (-8.1562, 52.3073) (-8.1426, 52.2801) (-8.1272, 52.254) (-8.1102, 52.2296) (-8.0923, 52.2066) (-8.0729, 52.1851) (-8.0521, 52.1653) (-8.0299, 52.1471) (-8.0066, 52.1302) (-7.9819, 52.1153) (-7.9562, 52.1016) (-7.9292, 52.0903) (-7.9016, 52.0802) (-7.8728, 52.0722) (-7.8431, 52.0659) (-7.8123, 52.0617) (-7.7805, 52.0585) (-7.759, 52.0584) (-7.7482, 52.0583) knots 0 0 0 0 0.044014 0.087434 0.130118 0.172554 0.214555 0.256298 0.298438 0.340849 0.382715 0.423924 0.464246 0.504074 0.543862 0.583567 0.623094 0.663229 0.703551 0.743938 0.784541 0.82575 0.867757 0.910745 0.954914 1 1 1 1
  spline S6 degree 3 poles (-7.755, 52.1916) (-7.7661, 52.1919) (-7.788, 52.1925) (-7.8202, 52.1971) (-7.8514, 52.2042) (-7.8811, 52.2149) (-7.9099, 52.2278) (-7.9371, 52.2444) (-7.9634, 52.2635) (-7.9881, 52.2854) (-8.0107, 52.3096) (-8.0306, 52.3354) (-8.0473, 52.3629) (-8.0613, 52.3917) (-8.0719, 52.422) (-8.0795, 52.4538) (-8.084, 52.487) (-8.0846, 52.5097) (-8.0849, 52.5213) knots 0 0 0 0 0.064207 0.126425 0.18768 0.248216 0.308305 0.369661 0.431699 0.495947 0.559758 0.622295 0.683911 0.745092 0.80674 0.869087 0.93329 1 1 1 1
  spline S7 degree 3 poles (-7.7925, 52.9416) (-7.807, 52.9413) (-7.8355, 52.9407) (-7.8773, 52.9347) (-7.9171, 52.9254) (-7.955, 52.9123) (-7.991, 52.8957) (-8.0247, 52.8748) (-8.0567, 52.8505) (-8.0864, 52.8225) (-8.1134, 52.7917) (-8.1371, 52.7586) (-8.1572, 52.7235) (-8.1734, 52.686) (-8.1863, 52.6467) (-8.1949, 52.605) (-8.2006, 52.5614) (-8.2012, 52.5315) (-8.2016, 52.5163) knots 0 0 0 0 0.065808 0.129394 0.190894 0.251281 0.310815 0.370371 0.430768 0.492881 0.555104 0.616067 0.677256 0.73826 0.800762 0.864778 0.931045 1 1 1 1
  spline S8 degree 3 poles (-8.0849, 52.5213) (-8.0847, 52.5317) (-8.0842, 52.5521) (-8.0803, 52.582) (-8.0735, 52.6102) (-8.064, 52.637) (-8.052, 52.6624) (-8.0374, 52.6863) (-8.0198, 52.7085) (-7.9997, 52.7289) (-7.9777, 52.7478) (-7.9534, 52.7639) (-7.9273, 52.7775) (-7.8997, 52.7891) (-7.87, 52.7975) (-7.8388, 52.8038) (-7.8057, 52.8075) (-7.783, 52.808) (-7.7714, 52.8083) knots 0 0 0 0 0.065351 0.127916 0.18836 0.247216 0.30563 0.36377 0.422661 0.482687 0.5433 0.604118 0.664965 0.727413 0.791468 0.858055 0.927037 1 1 1 1
  line L40 (-8.1516, 53.2583) -> (-7.7094, 53.2583)
  line L41 (-7.6182, 53.3916) -> (-8.1516, 53.3916)
  line L42 (-3.8449, 53.3916) -> (-3.8449, 53.2583)
  spline S9 degree 3 poles (-3.4858, 52.9416) (-3.5003, 52.9413) (-3.5289, 52.9407) (-3.5706, 52.9347) (-3.6105, 52.9254) (-3.6484, 52.9123) (-3.6843, 52.8957) (-3.7181, 52.8748) (-3.7501, 52.8505) (-3.7798, 52.8225) (-3.8067, 52.7917) (-3.8304, 52.7586) (-3.8505, 52.7235) (-3.8667, 52.686) (-3.8796, 52.6467) (-3.8882, 52.605) (-3.8939, 52.5614) (-3.8946, 52.5315) (-3.8949, 52.5163) knots 0 0 0 0 0.065808 0.129394 0.190894 0.251281 0.310815 0.370371 0.430768 0.492881 0.555104 0.616067 0.677256 0.73826 0.800762 0.864778 0.931045 1 1 1 1
  spline S10 degree 3 poles (-3.8949, 52.5163) (-3.8947, 52.5057) (-3.8942, 52.4847) (-3.8917, 52.4534) (-3.8869, 52.4228) (-3.8804, 52.3929) (-3.872, 52.3637) (-3.8619, 52.3351) (-3.8495, 52.3073) (-3.8359, 52.2801) (-3.8206, 52.254) (-3.8036, 52.2296) (-3.7856, 52.2066) (-3.7663, 52.1851) (-3.7454, 52.1653) (-3.7232, 52.1471) (-3.7, 52.1302) (-3.6752, 52.1153) (-3.6495, 52.1016) (-3.6225, 52.0903) (-3.5949, 52.0802) (-3.5662, 52.0722) (-3.5364, 52.0659) (-3.5056, 52.0617) (-3.4739, 52.0585) (-3.4524, 52.0584) (-3.4415, 52.0583) knots 0 0 0 0 0.044014 0.087434 0.130118 0.172554 0.214555 0.256298 0.298438 0.340849 0.382715 0.423924 0.464246 0.504074 0.543862 0.583567 0.623094 0.663229 0.703551 0.743938 0.784541 0.82575 0.867757 0.910745 0.954914 1 1 1 1
  spline S11 degree 3 poles (-3.7782, 52.5213) (-3.778, 52.5317) (-3.7775, 52.5521) (-3.7736, 52.582) (-3.7668, 52.6102) (-3.7574, 52.637) (-3.7454, 52.6624) (-3.7307, 52.6863) (-3.7131, 52.7085) (-3.693, 52.7289) (-3.671, 52.7478) (-3.6467, 52.7639) (-3.6206, 52.7775) (-3.5931, 52.7891) (-3.5634, 52.7975) (-3.5321, 52.8038) (-3.499, 52.8075) (-3.4763, 52.808) (-3.4647, 52.8083) knots 0 0 0 0 0.065351 0.127916 0.18836 0.247216 0.30563 0.36377 0.422661 0.482687 0.5433 0.604118 0.664965 0.727413 0.791468 0.858055 0.927037 1 1 1 1
  line L43 (-3.8449, 53.2583) -> (-3.4027, 53.2583)
  line L44 (-3.4027, 53.2583) -> (-3.3327, 52.9163)
  spline S12 degree 3 poles (-3.3327, 52.9163) (-3.3464, 52.9201) (-3.3731, 52.9275) (-3.4125, 52.9357) (-3.4498, 52.9406) (-3.4741, 52.9413) (-3.4858, 52.9416) knots 0 0 0 0 0.275068 0.532901 0.773973 1 1 1 1
  line L45 (-3.3116, 53.3916) -> (-3.8449, 53.3916)
  line L46 (-3.1782, 52.7416) -> (-3.3116, 53.3916)
  spline S13 degree 3 poles (-3.4647, 52.8083) (-3.4546, 52.808) (-3.4338, 52.8076) (-3.4019, 52.8043) (-3.3684, 52.799) (-3.3333, 52.7917) (-3.2967, 52.7822) (-3.2586, 52.7708) (-3.2188, 52.7572) (-3.192, 52.7469) (-3.1782, 52.7416) knots 0 0 0 0 0.102203 0.211023 0.3251 0.446502 0.573788 0.708901 0.850358 1 1 1 1
  spline S14 degree 3 poles (-3.4483, 52.1916) (-3.4594, 52.1919) (-3.4813, 52.1925) (-3.5136, 52.1971) (-3.5447, 52.2042) (-3.5744, 52.2149) (-3.6032, 52.2278) (-3.6304, 52.2444) (-3.6567, 52.2635) (-3.6814, 52.2854) (-3.704, 52.3096) (-3.724, 52.3354) (-3.7406, 52.3629) (-3.7546, 52.3917) (-3.7653, 52.422) (-3.7729, 52.4538) (-3.7773, 52.487) (-3.7779, 52.5097) (-3.7782, 52.5213) knots 0 0 0 0 0.064207 0.126425 0.18768 0.248216 0.308305 0.369661 0.431699 0.495947 0.559758 0.622295 0.683911 0.745092 0.80674 0.869087 0.93329 1 1 1 1
  arc A8 (-19.9782, 47.8916) -> (-19.8782, 47.7916) centre (-19.8782, 47.8916) ccw
  line L47 (-16.9525, 47.7916) -> (-19.8782, 47.7916)
  spline S15 degree 3 poles (-3.1616, 52.4249) (-3.1644, 52.4125) (-3.17, 52.3887) (-3.1821, 52.3552) (-3.1969, 52.3254) (-3.2145, 52.2988) (-3.2355, 52.2756) (-3.2595, 52.255) (-3.2863, 52.2363) (-3.3162, 52.2208) (-3.3477, 52.2075) (-3.3807, 52.1987) (-3.4142, 52.1925) (-3.4369, 52.1919) (-3.4483, 52.1916) knots 0 0 0 0 0.094687 0.181994 0.264377 0.34218 0.418618 0.496509 0.577369 0.661511 0.746733 0.831258 0.915206 1 1 1 1
  line L48 (-3.0449, 52.4249) -> (-3.1616, 52.4249)
  spline S16 degree 3 poles (-3.4415, 52.0583) (-3.4286, 52.0585) (-3.4031, 52.059) (-3.3657, 52.0643) (-3.3298, 52.0719) (-3.2956, 52.0832) (-3.2628, 52.0975) (-3.2318, 52.1155) (-3.2019, 52.1359) (-3.1742, 52.16) (-3.1485, 52.1864) (-3.1255, 52.215) (-3.105, 52.2453) (-3.0874, 52.2776) (-3.0723, 52.3117) (-3.0605, 52.3478) (-3.051, 52.3856) (-3.047, 52.4117) (-3.0449, 52.4249) knots 0 0 0 0 0.065421 0.128708 0.190236 0.250724 0.310637 0.370766 0.431615 0.493523 0.555883 0.617342 0.678668 0.740711 0.802985 0.866803 0.932347 1 1 1 1
  spline S17 degree 3 poles (-12.6064, 52.2856) (-12.5933, 52.3018) (-12.5671, 52.3339) (-12.5336, 52.386) (-12.505, 52.4404) (-12.4818, 52.4974) (-12.4637, 52.5569) (-12.4511, 52.6188) (-12.443, 52.6831) (-12.442, 52.7269) (-12.4416, 52.7491) knots 0 0 0 0 0.124329 0.247156 0.36878 0.490734 0.613614 0.738958 0.867311 1 1 1 1
  spline S18 degree 3 poles (-12.4416, 52.7491) (-12.4422, 52.7725) (-12.4433, 52.8185) (-12.4529, 52.886) (-12.4685, 52.9507) (-12.4905, 53.0125) (-12.5185, 53.0716) (-12.5531, 53.1276) (-12.5938, 53.1809) (-12.6404, 53.2307) (-12.6915, 53.2762) (-12.7462, 53.3162) (-12.8044, 53.3496) (-12.8655, 53.3774) (-12.93, 53.3988) (-12.9976, 53.4138) (-13.0683, 53.4231) (-13.1165, 53.4243) (-13.1411, 53.4249) knots 0 0 0 0 0.064558 0.127014 0.187955 0.248014 0.307748 0.368235 0.42947 0.492743 0.556258 0.618217 0.679655 0.741246 0.803415 0.866815 0.932328 1 1 1 1
  spline S19 degree 3 poles (-13.1338, 53.2916) (-13.1207, 53.2914) (-13.0948, 53.2911) (-13.0563, 53.2872) (-13.0185, 53.2817) (-12.9815, 53.2734) (-12.9452, 53.2631) (-12.9095, 53.2506) (-12.8749, 53.2353) (-12.8409, 53.2183) (-12.8083, 53.1991) (-12.7774, 53.1782) (-12.7485, 53.1558) (-12.7213, 53.1318) (-12.696, 53.1063) (-12.6727, 53.079) (-12.6514, 53.0501) (-12.6319, 53.0199) (-12.6143, 52.9885) (-12.5996, 52.9558) (-12.5866, 52.9223) (-12.5763, 52.8877) (-12.5682, 52.8522) (-12.5626, 52.8158) (-12.5587, 52.7784) (-12.5584, 52.7531) (-12.5582, 52.7403) knots 0 0 0 0 0.043955 0.087502 0.130463 0.172752 0.215403 0.25765 0.300153 0.343121 0.385925 0.427686 0.468818 0.509492 0.549883 0.58998 0.630405 0.670869 0.711384 0.751627 0.791776 0.832459 0.873319 0.914543 0.956924 1 1 1 1
  spline S20 degree 3 poles (-12.5582, 52.7403) (-12.5587, 52.7211) (-12.5596, 52.6833) (-12.5678, 52.6281) (-12.5803, 52.5752) (-12.5989, 52.5249) (-12.6219, 52.4766) (-12.651, 52.4312) (-12.6846, 52.388) (-12.7234, 52.3479) (-12.7659, 52.3113) (-12.8114, 52.2791) (-12.86, 52.2522) (-12.9111, 52.2299) (-12.9649, 52.2127) (-13.0215, 52.2006) (-13.0808, 52.1927) (-13.1212, 52.192) (-13.1418, 52.1916) knots 0 0 0 0 0.064323 0.12629 0.186726 0.246146 0.305576 0.365429 0.426326 0.48884 0.551725 0.613919 0.675484 0.737334 0.800229 0.864502 0.931041 1 1 1 1
  spline S21 degree 3 poles (-13.1426, 52.0583) (-13.1286, 52.0584) (-13.101, 52.0585) (-13.0602, 52.0617) (-13.0204, 52.0659) (-12.9819, 52.0723) (-12.9443, 52.0799) (-12.9081, 52.09) (-12.8728, 52.1013) (-12.8387, 52.1147) (-12.8056, 52.1297) (-12.7737, 52.1467) (-12.743, 52.1656) (-12.7132, 52.1858) (-12.6848, 52.2081) (-12.6574, 52.2321) (-12.631, 52.2578) (-12.6146, 52.2763) (-12.6064, 52.2856) knots 0 0 0 0 0.069663 0.13775 0.203917 0.26878 0.332414 0.394754 0.45618 0.516996 0.577396 0.637198 0.696999 0.756756 0.816554 0.876948 0.938132 1 1 1 1
  spline S22 degree 3 poles (-13.1418, 52.1916) (-13.1645, 52.1922) (-13.2092, 52.1934) (-13.2747, 52.2039) (-13.3374, 52.2209) (-13.3973, 52.2446) (-13.4543, 52.2755) (-13.5084, 52.3129) (-13.5596, 52.3572) (-13.5904, 52.391) (-13.6062, 52.4083) knots 0 0 0 0 0.128515 0.252949 0.374755 0.49594 0.617181 0.740909 0.867811 1 1 1 1
  spline S23 degree 3 poles (-13.7082, 52.3309) (-13.7, 52.3203) (-13.6836, 52.2992) (-13.6571, 52.2693) (-13.6291, 52.2413) (-13.5995, 52.2153) (-13.5687, 52.1907) (-13.536, 52.1683) (-13.5018, 52.1477) (-13.4664, 52.1289) (-13.4297, 52.1123) (-13.3919, 52.098) (-13.3529, 52.0857) (-13.3129, 52.0756) (-13.2718, 52.0676) (-13.2297, 52.0624) (-13.1865, 52.0587) (-13.1574, 52.0584) (-13.1426, 52.0583) knots 0 0 0 0 0.061674 0.123053 0.183475 0.243727 0.304279 0.364863 0.425946 0.487391 0.54922 0.611144 0.673529 0.736961 0.800785 0.866013 0.932101 1 1 1 1
  line L49 (-13.6062, 52.4083) -> (-13.7082, 52.3309)
  spline S24 degree 3 poles (-13.6062, 53.0749) (-13.5989, 53.0836) (-13.5844, 53.1008) (-13.5611, 53.125) (-13.5369, 53.1477) (-13.5117, 53.169) (-13.485, 53.1881) (-13.4576, 53.206) (-13.4289, 53.2221) (-13.3892, 53.2416) (-13.3374, 53.2619) (-13.2721, 53.279) (-13.2039, 53.2898) (-13.1574, 53.291) (-13.1338, 53.2916) knots 0 0 0 0 0.063163 0.125475 0.187121 0.248294 0.309295 0.36985 0.430973 0.492456 0.616148 0.740844 0.868183 1 1 1 1
  line L50 (-13.7082, 53.153) -> (-13.6062, 53.0749)
  spline S25 degree 3 poles (-13.1411, 53.4249) (-13.156, 53.4247) (-13.1856, 53.4244) (-13.2293, 53.4209) (-13.2719, 53.4152) (-13.3133, 53.4073) (-13.3539, 53.3976) (-13.3932, 53.3849) (-13.4315, 53.3704) (-13.4685, 53.3537) (-13.5041, 53.335) (-13.5383, 53.3144) (-13.5708, 53.292) (-13.6018, 53.268) (-13.6308, 53.2418) (-13.6587, 53.2143) (-13.6844, 53.1845) (-13.7003, 53.1635) (-13.7082, 53.153) knots 0 0 0 0 0.068548 0.135683 0.201215 0.265682 0.329267 0.392395 0.45507 0.517127 0.57879 0.63974 0.700192 0.759806 0.819628 0.879355 0.939512 1 1 1 1
  line L51 (-15.0825, 56.2076) -> (-14.9908, 57.6416)
  line L52 (-6.3916, 52.9916) -> (-6.2749, 52.9916)
  line L53 (-6.2249, 52.0916) -> (-6.7291, 52.6296)
  spline S26 degree 3 poles (-6.2749, 52.9916) (-6.2757, 53.0071) (-6.2772, 53.0375) (-6.2842, 53.0818) (-6.2942, 53.1241) (-6.3083, 53.1642) (-6.3259, 53.2023) (-6.347, 53.2384) (-6.3719, 53.2722) (-6.4002, 53.3034) (-6.431, 53.3321) (-6.4641, 53.3568) (-6.499, 53.3778) (-6.5354, 53.3952) (-6.5738, 53.4084) (-6.6139, 53.4181) (-6.6558, 53.424) (-6.6843, 53.4246) (-6.6989, 53.4249) knots 0 0 0 0 0.068791 0.135103 0.198979 0.261904 0.323495 0.385195 0.446969 0.509765 0.572251 0.633405 0.693251 0.752583 0.812579 0.873275 0.93555 1 1 1 1
  line L54 (-6.8286, 52.5721) -> (-6.5033, 52.2249)
  line L55 (-7.1082, 52.0916) -> (-6.2249, 52.0916)
  spline S27 degree 3 poles (-6.7291, 52.6296) (-6.7413, 52.6424) (-6.7649, 52.667) (-6.7983, 52.703) (-6.8282, 52.7363) (-6.855, 52.767) (-6.8779, 52.7954) (-6.8983, 52.8208) (-6.9147, 52.8441) (-6.9324, 52.8711) (-6.9495, 52.9041) (-6.9643, 52.9444) (-6.9733, 52.9859) (-6.9744, 53.0139) (-6.9749, 53.028) knots 0 0 0 0 0.110803 0.212829 0.306101 0.390647 0.466924 0.534481 0.593587 0.644557 0.7362 0.825024 0.911986 1 1 1 1
  spline S28 degree 3 poles (-6.9749, 53.028) (-6.9747, 53.0369) (-6.9742, 53.0544) (-6.9701, 53.08) (-6.9639, 53.1048) (-6.955, 53.1286) (-6.9433, 53.1515) (-6.929, 53.1732) (-6.9125, 53.1943) (-6.8934, 53.214) (-6.8725, 53.2321) (-6.8503, 53.2481) (-6.8269, 53.2615) (-6.8023, 53.2725) (-6.7766, 53.2811) (-6.7497, 53.2871) (-6.7217, 53.2908) (-6.7026, 53.2913) (-6.6929, 53.2916) knots 0 0 0 0 0.061965 0.122122 0.180988 0.239933 0.299906 0.359989 0.421776 0.486576 0.551535 0.615018 0.677259 0.73973 0.80305 0.866495 0.931973 1 1 1 1
  line L56 (-6.5033, 52.2249) -> (-7.1082, 52.2249)
  spline S29 degree 3 poles (-7.0916, 53.0385) (-7.0909, 53.0204) (-7.0897, 52.9845) (-7.079, 52.9317) (-7.0624, 52.8806) (-7.0423, 52.8395) (-7.0221, 52.8063) (-7.0039, 52.779) (-6.9825, 52.7497) (-6.9577, 52.7183) (-6.9301, 52.6847) (-6.8992, 52.6488) (-6.865, 52.6111) (-6.841, 52.5854) (-6.8286, 52.5721) knots 0 0 0 0 0.098702 0.195672 0.292422 0.391343 0.444462 0.504229 0.570352 0.642546 0.722288 0.807921 0.90047 1 1 1 1
  spline S30 degree 3 poles (-6.6989, 53.4249) (-6.7131, 53.4246) (-6.7411, 53.4239) (-6.782, 53.4183) (-6.8209, 53.4095) (-6.8578, 53.3971) (-6.8924, 53.3805) (-6.9248, 53.3605) (-6.9556, 53.3374) (-6.9833, 53.3102) (-7.0088, 53.2811) (-7.0307, 53.2501) (-7.0495, 53.2181) (-7.0652, 53.1848) (-7.0767, 53.1499) (-7.0855, 53.114) (-7.0904, 53.0766) (-7.0912, 53.0513) (-7.0916, 53.0385) knots 0 0 0 0 0.069475 0.136517 0.200789 0.26383 0.325735 0.387291 0.449509 0.512968 0.576275 0.63758 0.697903 0.757172 0.816599 0.876653 0.93729 1 1 1 1
  line L57 (-7.1082, 52.2249) -> (-7.1082, 52.0916)
  line L58 (-7.4849, 52.7416) -> (-7.6182, 53.3916)
  line L59 (-7.7094, 53.2583) -> (-7.6393, 52.9163)
  spline S31 degree 3 poles (-7.7482, 52.0583) (-7.7352, 52.0585) (-7.7098, 52.059) (-7.6724, 52.0643) (-7.6365, 52.0719) (-7.6023, 52.0832) (-7.5694, 52.0975) (-7.5385, 52.1155) (-7.5085, 52.1359) (-7.4808, 52.16) (-7.4552, 52.1864) (-7.4322, 52.215) (-7.4117, 52.2453) (-7.3941, 52.2776) (-7.379, 52.3117) (-7.3672, 52.3478) (-7.3577, 52.3856) (-7.3536, 52.4117) (-7.3516, 52.4249) knots 0 0 0 0 0.065421 0.128708 0.190236 0.250724 0.310637 0.370766 0.431615 0.493523 0.555883 0.617342 0.678668 0.740711 0.802985 0.866803 0.932347 1 1 1 1
  spline S32 degree 3 poles (-7.4682, 52.4249) (-7.4711, 52.4125) (-7.4766, 52.3887) (-7.4887, 52.3552) (-7.5035, 52.3254) (-7.5212, 52.2988) (-7.5422, 52.2756) (-7.5661, 52.255) (-7.593, 52.2363) (-7.6229, 52.2208) (-7.6544, 52.2075) (-7.6873, 52.1987) (-7.7209, 52.1925) (-7.7436, 52.1919) (-7.755, 52.1916) knots 0 0 0 0 0.094687 0.181994 0.264377 0.34218 0.418618 0.496509 0.577369 0.661511 0.746733 0.831258 0.915206 1 1 1 1
  spline S33 degree 3 poles (-7.7714, 52.8083) (-7.7613, 52.808) (-7.7405, 52.8076) (-7.7086, 52.8043) (-7.675, 52.799) (-7.64, 52.7917) (-7.6034, 52.7822) (-7.5652, 52.7708) (-7.5255, 52.7572) (-7.4987, 52.7469) (-7.4849, 52.7416) knots 0 0 0 0 0.102203 0.211023 0.3251 0.446502 0.573788 0.708901 0.850358 1 1 1 1
  spline S34 degree 3 poles (-7.6393, 52.9163) (-7.6531, 52.9201) (-7.6798, 52.9275) (-7.7191, 52.9357) (-7.7565, 52.9406) (-7.7807, 52.9413) (-7.7925, 52.9416) knots 0 0 0 0 0.275068 0.532901 0.773973 1 1 1 1
  line L60 (-7.3516, 52.4249) -> (-7.4682, 52.4249)
  line L61 (-7.4525, 47.7916) -> (-12.704, 47.7916)
  arc A9 (-7.099, 47.6451) -> (-7.4525, 47.7916) centre (-7.4525, 47.2916) ccw
  line L62 (-6.7747, 47.3209) -> (-7.099, 47.6451)
  arc A10 (-6.7747, 47.3209) -> (-6.704, 47.2916) centre (-6.704, 47.3916) ccw
  arc A11 (-10.6318, 57.6123) -> (-10.7025, 57.6416) centre (-10.7025, 57.5416) ccw
  line L63 (-10.6318, 57.6123) -> (-10.3075, 57.288)
  arc A12 (-10.3075, 57.288) -> (-9.954, 57.1416) centre (-9.954, 57.6416) ccw
  line L64 (-9.954, 57.1416) -> (-0.2782, 57.1416)
  arc A13 (-0.1782, 57.0416) -> (-0.2782, 57.1416) centre (-0.2782, 57.0416) ccw
  line L65 (-0.1782, 57.0416) -> (-0.1782, 47.8916)
  circle A14 centre (-5.3282, 49.8416) radius 1.25
  arc A15 (-0.2782, 47.7916) -> (-0.1782, 47.8916) centre (-0.2782, 47.8916) ccw
  line L66 (-0.2782, 47.7916) -> (-3.204, 47.7916)
  arc A16 (-3.204, 47.7916) -> (-3.5575, 47.6451) centre (-3.204, 47.2916) ccw
  arc A17 (-3.9525, 47.2916) -> (-3.8818, 47.3209) centre (-3.9525, 47.3916) ccw